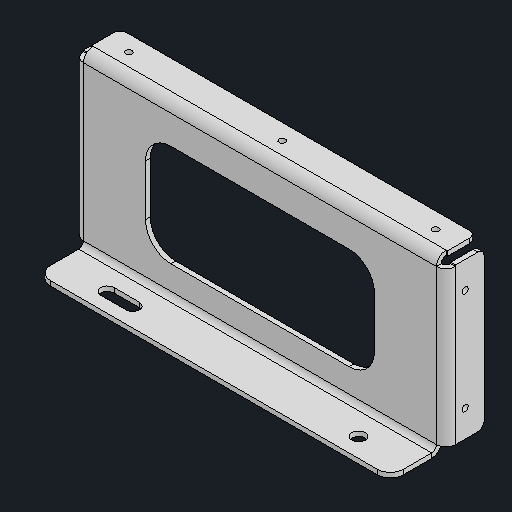
# Autodesk Inventor part: 5th Wheel Hitch Part 3
Saved by Autodesk Inventor 2025.1 (Build 291241000, 241)
## iProperties
Created: 2026-02-23
Part Number: 5th Wheel Hitch Part 3
Material: Generic
Document SubType Name: Sheet Metal
Designer: Desktop -24
Density: 1 g/cm^3
Sheet Metal Rule: Default
Appearance: Default
Author: Desktop -24
Autodesk Inventor part; units mm, degrees
note: some values were not read from the file. Chosen so that the rebuilt part matches the saved one: corner form of "Plate5".
ref_plane "YZ Plane" through (0, 0, 0) normal (1, 0, 0) x (0, 1, 0)
ref_plane "XZ Plane" through (0, 0, 0) normal (0, 1, 0) x (-1, 0, 0)
ref_plane "XY Plane" through (0, 0, 0) normal (0, 0, 1) x (1, 0, 0)
sketch "Sketch9" plane through (0, 0, 0) normal (0, 0, 1) x (1, 0, 0)
  line L0 (-371.475, 0) -> (371.475, 0)
  line L1 (371.475, 0) -> (371.475, -327.0319)
  line L2 (371.475, -327.0319) -> (-371.475, -327.0319)
  line L3 (-371.475, -327.0319) -> (-371.475, 0)
  point P0 (0, 0)
  point P1 (0, 0)
  dimension "d62" = 742.95
  dimension "d83" = 327.0319
  measures "d62" distance of L0.start L0.end
  measures "d83" distance of L0.end L1.end
extrude "Plate4" add sketch "Sketch9" along normal blind 9.525
sketch "Sketch10" plane through (361.95, -327.0319, 9.525) normal (1, 0, 0) x (0, 1, 0)
  line L0 (327.0319, 0) -> (0, 0)
  line L1 (0, 0) -> (0, -76.2)
  line L2 (0, -76.2) -> (327.0319, -76.2)
  line L3 (327.0319, -76.2) -> (327.0319, 0)
  constraints: 6 end point, 1 horizontal, 1 perpendicular, 1 vertical
edge flange "Flange3" height 76.2 angle 90 thickness 9.525 bend radius 9.525 thickness toward (1, 0, 0) relief tear relief width 9.525 relief depth 4.7625 corner gap 9.525 corner form 2 edges at (371.475, -163.5159, 0) (-371.475, -163.5159, 0) (0, 0, 0) wall of the first edge with corners at (361.95, 0, 9.525) (361.95, -327.0319, 9.525) (361.95, -327.0319, -66.675) (361.95, 0, -66.675)
bend "Bend3"
corner "Corner3"
sketch "Sketch11" plane through (352.425, -336.5569, 19.05) normal (0, -1, 0) x (1, 0, 0)
  line L0 (-704.85, 0) -> (0, 0)
  line L1 (0, 0) -> (0, 82.55)
  line L2 (0, 82.55) -> (-704.85, 82.55)
  line L3 (-704.85, 82.55) -> (-704.85, 0)
  constraints: 6 end point, 1 horizontal, 1 perpendicular, 1 vertical
edge flange "Flange4" height 101.6 angle 90 thickness 9.525 bend radius 9.525 thickness toward (0, -1, 0) relief tear relief width 9.525 relief depth 4.7625 edges at (0, -327.0319, 9.525) wall of the first edge with corners at (-352.425, -336.5569, 19.05) (352.425, -336.5569, 19.05) (352.425, -336.5569, 101.6) (-352.425, -336.5569, 101.6)
bend "Bend4"
corner "Corner4"
sketch "Sketch12" plane through (0, 0, 9.525) normal (0, 0, 1) x (1, 0, 0)
  line L0 (-228.6, -279.4) -> (228.6, -279.4)
  line L1 (228.6, -279.4) -> (228.6, -76.2)
  line L2 (228.6, -76.2) -> (-228.6, -76.2)
  line L3 (-228.6, -76.2) -> (-228.6, -279.4)
  line L4 (-228.6, -279.4) -> (228.6, -76.2) construction
  line L5 (228.6, -279.4) -> (-228.6, -76.2) construction
  line L6 (-352.425, 0) -> (352.425, 0) projected
  point P0 (0, 0)
  point P1 (0, -177.8)
  dimension "d84" = 457.2
  dimension "d85" = 76.2
  dimension "d86" = 203.2
  constraints: 12 end point, 2 midpoint, 2 parallel, 1 horizontal, 1 perpendicular
  measures "d84" distance of L1.end L2.end
  measures "d85" distance between parallel lines of L2 L6
  measures "d86" distance of L2.end L0.start
extrude "Cut2" cut sketch "Sketch12" against normal blind 9.525
fillet "Corner Round5" radius 50.8 4 edges at (228.6, -76.2, 4.7625) (-228.6, -76.2, 4.7625) (228.6, -279.4, 4.7625) (-228.6, -279.4, 4.7625)
fillet "Corner Round6" radius 25.4 2 edges at (352.425, -341.3194, 101.6) (-352.425, -341.3194, 101.6)
fillet "Corner Round7" radius 12.7 6 edges at (355.2148, -4.7625, -66.675) (-355.2148, -4.7625, -66.675) (366.7125, -327.0319, -66.675) (366.7125, -16.2602, -66.675) (-366.7125, -327.0319, -66.675) (-366.7125, -16.2602, -66.675)
sketch "Sketch13" plane through (-371.475, -327.0319, -9.525) normal (-1, 0, 0) x (0, 0, 1)
  line L0 (-19.05, 256.9859) -> (-19.05, 53.7859)
  line L1 (-57.15, 12.7) -> (-57.15, 298.0717) construction
  line L2 (19.05, 307.9819) -> (19.05, 0) projected
  point P0 (9.525, 327.0319)
  point P1 (-57.15, 155.3859)
  point P2 (-19.05, 155.3859)
  dimension "d92" = 38.1
  dimension "d93" = 203.2
  constraints: 2 end point, 2 midpoint, 1 horizontal alignment, 1 vertical
  measures "d92" distance between parallel lines of L2 L0
  measures "d93" distance of L0.start L0.end
hole "Hole1" at (-371.475, -70.046, -28.575) at (-371.475, -273.246, -28.575) direction (1, 0, 0) diameter 12.7 end through all
sketch "Sketch14" plane through (-352.425, -336.5569, 19.05) normal (0, 1, 0) x (1, 0, 0)
  circle A0 centre (603.25, -44.45) radius 13.335
  line L0 (704.85, -57.15) -> (704.85, 0) projected
  line L1 (101.6, -44.45) -> (152.4, -44.45) construction
  line L2 (101.6, -31.115) -> (152.4, -31.115)
  line L3 (152.4, -57.785) -> (101.6, -57.785)
  arc A1 (101.6, -31.115) -> (101.6, -57.785) centre (101.6, -44.45) ccw
  arc A2 (152.4, -57.785) -> (152.4, -31.115) centre (152.4, -44.45) ccw
  line L4 (0, -57.15) -> (0, 0) projected
  line L5 (25.4, -82.55) -> (679.45, -82.55) projected
  point P0 (352.425, 19.05)
  point P1 (127, -44.45)
  point P2 (0, -28.575)
  dimension "d101" = 101.6
  dimension "d103" = 101.6
  dimension "d104" = 50.8
  dimension "d105" = 38.1
  dimension "d106" = 13.335
  dimension "d107" = 26.67
  constraints: 8 end point, 4 point on circle, 4 tangent, 3 centre point, 2 midpoint, 1 horizontal, 1 horizontal alignment, 1 parallel
  measures "d101" distance from line of L0 A0.centre
  measures "d103" horizontal distance of point (0, -28.575) L1.start
  measures "d104" distance of L1.start L1.end
  measures "d105" distance between parallel lines of L5 L1
  measures "d106" radius of A2
  measures "d107" diameter of A0
extrude "Cut3" cut sketch "Sketch14" against normal blind 9.525
sketch "Sketch15" plane through (-352.425, 0, -9.525) normal (0, 1, 0) x (1, 0, 0)
  line L0 (46.0375, 25.4) -> (658.8125, 25.4)
  line L1 (9.9102, 57.15) -> (694.9398, 57.15) projected
  line L2 (-2.7898, 0) -> (-2.7898, 44.45) projected
  line L3 (707.6398, 44.45) -> (707.6398, 0) projected
  point P0 (352.425, -9.525)
  point P1 (-2.7898, 22.225)
  point P2 (707.6398, 22.225)
  point P3 (352.425, 25.4)
  dimension "d110" = 31.75
  dimension "d111" = 48.8273
  dimension "d112" = 48.8273
  constraints: 3 midpoint, 2 end point, 1 horizontal
  measures "d110" distance between parallel lines of L0 L1
  measures "d111" horizontal distance of point (-2.79, 22.225) L0.start
  measures "d112" horizontal distance of point (707.64, 22.225) L0.end
hole "Hole2" at (-306.3875, 0, -34.925) at (306.3875, 0, -34.925) at (0, 0, -34.925) direction (0, -1, 0) diameter 12.7 end through all
equation "\"d87\" = Thickness"
equation "\"d99\" = Thickness"
equation "\"d103\" = d101"
equation "\"d107\" = 2 * d106"
equation "\"d108\" = Thickness"
equation "\"d61\" = Thickness"
equation "\"d63\" = BendReliefWidth"
equation "\"d64\" = BendReliefDepth"
equation "\"d65\" = MinimumRemnant"
equation "\"d66\" = TransitionRadius"
equation "\"d69\" = BendRadius"
equation "\"d70\" = CornerReliefSize"
equation "\"d71\" = GapSize"
equation "\"d72\" = JacobiRadiusSize"
equation "\"d73\" = BendReliefWidth"
equation "\"d74\" = BendReliefDepth"
equation "\"d75\" = MinimumRemnant"
equation "\"d76\" = TransitionRadius"
equation "\"d79\" = BendRadius"
equation "\"d80\" = CornerReliefSize"
equation "\"d81\" = GapSize"
equation "\"d82\" = JacobiRadiusSize"
equation "\"d111\" = d112"
equation "\"BendRadius\" = Thickness"
equation "\"BendReliefWidth\" = Thickness"
equation "\"BendReliefDepth\" = 0.5 * Thickness"
equation "\"CornerReliefSize\" = 4 * Thickness"
equation "\"MinimumRemnant\" = 2 * Thickness"
equation "\"TransitionRadius\" = BendRadius"
equation "\"JacobiRadiusSize\" = BendRadius"
equation "\"GapSize\" = Thickness"
equation "\"Thickness\" = 9.525"
body "Solid2"
